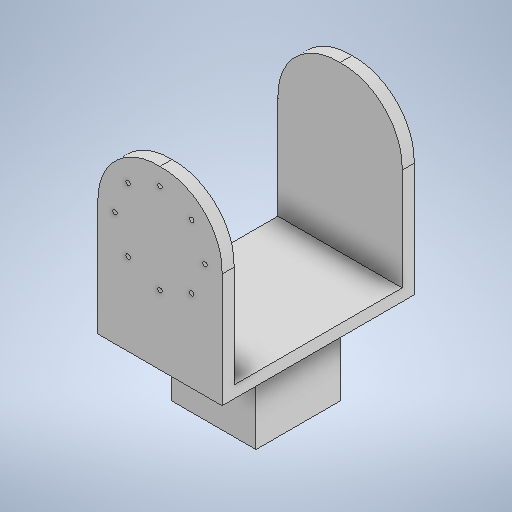
# Autodesk Inventor part: horn_connector
Saved by Autodesk Inventor 2025 (Build 290162000, 162)
## iProperties
Created: 2024-05-26
Part Number: horn_connector
Material: Generic
Document SubType Name: Modeling
Designer: hifzh
Density: 1 g/cm^3
Appearance: Default
Author: hifzh
Autodesk Inventor part; units mm, degrees
ref_plane "YZ Plane" through (0, 0, 0) normal (1, 0, 0) x (0, 1, 0)
ref_plane "XY Plane" through (0, 0, 0) normal (0, 0, 1) x (1, 0, 0)
sketch "Sketch1" plane through (0, 0, 0) normal (0, 0, 1) x (1, 0, 0)
  line L0 (20.705, -38) -> (-20.705, -38)
  arc A0 (0, 20.704) -> (-20.705, 0) centre (-0.7179, 0.7169) ccw
  arc A1 (20.705, 0) -> (0, 20.704) centre (0.7179, 0.7169) ccw
  line L1 (-20.705, 0) -> (-20.705, -38)
  line L2 (20.705, 0) -> (20.705, -38)
  point P0 (0, 0)
  point P1 (0, -38)
  dimension "d3" = 20
  dimension "d4" = 20
  constraints: 6 end point, 4 point on circle, 2 centre point, 1 midpoint, 1 parallel, 1 vertical, 1 vertical alignment
  measures "d3" radius of A0
  measures "d4" radius of A1
extrude "Extrusion1" add sketch "Sketch1" along normal blind 64
ref_plane "Work Plane1" through (0, 0, 4) normal (0, 0, -1) x (-1, 0, 0)
ref_plane "Work Plane2" through (0, 0, 60) normal (0, 0, -1) x (-1, 0, 0)
ref_plane "Work Plane3" through (0, 0, 32) normal (0, 0, -1) x (-1, 0, 0)
sketch "Sketch2" plane through (0, 0, 32) normal (0, 0, -1) x (-1, 0, 0)
  arc A0 (0, 20.704) -> (-20.705, 0) centre (-0.7179, 0.7169) ccw projected
  line L0 (-20.705, -38) -> (-20.705, 0) projected
  arc A1 (0, 20.704) -> (-20.705, 0) centre (-0.7179, 0.7169) ccw
  arc A2 (20.705, 0) -> (0, 20.704) centre (0.7179, 0.7169) ccw projected
  arc A3 (20.705, 0) -> (0, 20.704) centre (0.7179, 0.7169) ccw
  line L1 (20.705, 0) -> (20.705, -38) projected
  line L2 (20.705, 0) -> (20.705, -34)
  line L3 (20.705, -34) -> (-20.705, -34)
  point P0 (0, 0)
  dimension "d10" = 20
  dimension "d11" = 20
  dimension "d12" = 34
  constraints: 4 end point, 4 point on circle, 2 centre point, 2 point on line, 1 perpendicular
  measures "d10" radius of A1
  measures "d11" radius of A3
  measures "d12" distance of L1.start L2.end
extrude "Extrusion2" cut sketch "Sketch2" along normal mid plane 56
sketch "Sketch3" plane through (0, 0, 60) normal (0, 0, -1) x (-1, 0, 0)
  circle A0 centre (0, 0) radius 17.705
  circle A1 centre (0, 0) radius 15
  circle A2 centre (0, 15) radius 0.75
  circle A3 centre (-10.6066, 10.6066) radius 0.75
  circle A4 centre (-15, 0) radius 0.75
  circle A5 centre (-10.6066, -10.6066) radius 0.75
  circle A6 centre (0, -15) radius 0.75
  circle A7 centre (10.6066, -10.6066) radius 0.75
  circle A8 centre (15, 0) radius 0.75
  circle A9 centre (10.6066, 10.6066) radius 0.75
  dimension "d16" = 30
  dimension "d15" = 35.41
  dimension "d17" = 1.5
  dimension "d20" = 360
  constraints: 9 centre point, 2 coincident, 1 vertical alignment, 19 other
  measures "d15" diameter of A0
  measures "d17" diameter of A2
extrude "Extrusion3" cut sketch "Sketch3" against normal blind 4 contours A1 A8 | A1 A8 | A9 A1 | A1 A9 | A7 A1 | A1 A7 | A2 A1 | A1 A2 | A6 A1 | A1 A6 | A3 A1 | A1 A3 | A5 A1 | A1 A5 | A4 A1 | A1 A4
sketch "Sketch4" plane through (0, 0, 60) normal (0, 0, -1) x (-1, 0, 0)
  circle A0 centre (0, 0) radius 17.705
  dimension "d24" = 35.41
  constraints: 1 centre point, 1 coincident
  measures "d24" diameter of A0
extrude "Extrusion4" cut sketch "Sketch4" against normal blind 1.5
ref_plane "Work Plane4" through (0, -38, 0) normal (0, 1, 0) x (-1, 0, 0)
sketch "Sketch5" plane through (-20.705, -38, 0) normal (0, -1, 0) x (1, 0, 0)
  line L0 (34.705, 46) -> (6.705, 46)
  line L1 (6.705, 46) -> (6.705, 18)
  line L2 (6.705, 18) -> (34.705, 18)
  line L3 (34.705, 18) -> (34.705, 46)
  line L4 (30.705, 42) -> (10.705, 42)
  line L5 (10.705, 42) -> (10.705, 22)
  line L6 (10.705, 22) -> (30.705, 22)
  line L7 (30.705, 22) -> (30.705, 42)
  line L8 (0, 0) -> (41.41, 0) projected
  line L9 (0, 0) -> (0, 64) projected
  line L10 (41.41, 0) -> (41.41, 64) projected
  point P0 (20.705, 0)
  point P1 (20.705, 18)
  point P2 (20.705, 22)
  point P3 (34.705, 32)
  point P4 (41.41, 32)
  dimension "d28" = 20
  dimension "d29" = 28
  dimension "d30" = 20
  dimension "d31" = 28
  dimension "d32" = 18
  dimension "d33" = 4
  dimension "d34" = 4
  dimension "d35" = 41.41
  dimension "d36" = 6.705
  constraints: 16 end point, 4 midpoint, 4 parallel, 2 horizontal, 2 perpendicular
  measures "d28" distance of L5.end L6.end
  measures "d29" distance of L1.end L2.end
  measures "d30" distance of L4.end L5.end
  measures "d31" distance of L0.end L1.end
  measures "d32" distance from line of point (20.705, 18) L8
  measures "d33" distance from line of L2 point (20.705, 22)
  measures "d34" distance between parallel lines of L1 L5
  measures "d35" distance between parallel lines of L9 L10
  measures "d36" distance of point (34.705, 32) point (41.41, 32)
extrude "Extrusion5" add sketch "Sketch5" along normal blind 25
body "Solid1"
